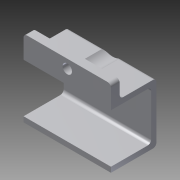
# Autodesk Inventor part: capot
Saved by Autodesk Inventor 2014 SP2 (Build 180246200, 246)
## iProperties
Created: 2015-03-19
Part Number: capot
Material: Plastique ABS
Document SubType Name: Modeling
Designer: sd
Density: 1.06 g/cm^3
Appearance: Lisse - Blanc
Mass: 7.9235 g
Surface Area: 23.98 cm^2
Volume: 7.475 cm^3
Author: sd
Autodesk Inventor part; units mm, degrees
ref_plane "YZ Plane" through (0, 0, 0) normal (1, 0, 0) x (0, 1, 0)
ref_plane "XZ Plane" through (0, 0, 0) normal (0, 1, 0) x (-1, 0, 0)
ref_plane "XY Plane" through (0, 0, 0) normal (0, 0, 1) x (1, 0, 0)
sketch "Esquisse1" plane through (0, 0, 0) normal (0, 1, 0) x (-1, 0, 0)
  line L0 (-12.5, 11) -> (12.5, 11)
  line L1 (12.5, 11) -> (12.5, -11)
  line L2 (12.5, -11) -> (-12.5, -11)
  line L3 (-12.5, -11) -> (-12.5, 11)
  point P0 (0, 0)
  dimension "d0" = 25
  dimension "d1" = 22
  dimension "d2" = 11
  dimension "d3" = 12.5
  constraints: 8 end point, 2 parallel, 1 horizontal, 1 perpendicular
  measures "d0" distance of L0.start L0.end
  measures "d1" distance of L2.end L0.start
  measures "d2" vertical distance of point (0, 0) L0.start
  measures "d3" horizontal distance of point (0, 0) L0.start
extrude "Extrusion1" add sketch "Esquisse1" along normal blind 13
sketch "Esquisse2" plane through (0, 13, 0) normal (0, 1, 0) x (1, 0, 0)
  line L0 (-12.5, 11) -> (-12.5, -11) projected
  line L1 (-12.5, -6) -> (12.5, -6)
  line L2 (12.5, -6) -> (12.5, -11)
  line L3 (12.5, -11) -> (-12.5, -11)
  line L4 (-12.5, -11) -> (-12.5, -6)
  point P0 (0, 0)
  dimension "d6" = 5
  constraints: 8 end point, 2 parallel, 1 horizontal, 1 perpendicular, 1 point on line
  measures "d6" distance of L3.end L1.start
extrude "Extrusion3" cut sketch "Esquisse2" against normal blind 10.5
fillet "Congé2" radius 1 1 edges at (0, 2.5, 6)
sketch "Esquisse4" plane through (0, 13, 0) normal (0, 1, 0) x (1, 0, 0)
  circle A0 centre (0, -8.5) radius 3.5
  line L0 (12.5, -11) -> (-12.5, -11) projected
  point P0 (12.5, -6)
  point P1 (0, 0)
  dimension "d11" = 7
  dimension "d12" = 2.5
  dimension "d13" = 5
  constraints: 1 centre point
  measures "d11" diameter of A0
  measures "d12" distance from line of L0 A0.centre
  measures "d13" distance of L0.start point (12.5, -6)
extrude "Extrusion4" cut sketch "Esquisse4" against normal blind 10.5
sketch "Esquisse6" plane through (0, 0, 0) normal (0, -1, 0) x (1, 0, 0)
  line L0 (-12.5, 11) -> (-12.5, -11) projected
  line L1 (-12.5, -11) -> (12.5, -11) projected
  line L2 (12.5, -11) -> (12.5, 11) projected
  line L3 (-12.5, -9.5) -> (12.5, -9.5)
  line L4 (12.5, -9.5) -> (12.5, 4.5)
  line L5 (12.5, 4.5) -> (-12.5, 4.5)
  line L6 (-12.5, 4.5) -> (-12.5, -9.5)
  point P0 (0, 0)
  dimension "d17" = 0
  dimension "d18" = 0
  dimension "d19" = 1.5
  dimension "d20" = 6.5
  constraints: 8 end point, 2 parallel, 1 horizontal, 1 perpendicular
  measures "d17" distance between parallel lines of L0 L6
  measures "d18" distance between parallel lines of L2 L4
  measures "d19" distance between parallel lines of L1 L3
  measures "d20" distance of L5.end L0.start
extrude "Extrusion5" cut sketch "Esquisse6" against normal blind 11.5 contours L5 L2 L3 L0
fillet "Congé3" radius 1 2 edges at (-12.5, 1.25, 11) (12.5, 1.25, 11)
fillet "Congé4" radius 1 5 edges at (0, 11.5, -9.5) (0, 13, -11) (0, 11.5, 4.5) (-7.4747, 13, 6) (7.4747, 13, 6)
sketch "Esquisse7" plane through (0, 2.5, 0) normal (0, 1, 0) x (1, 0, 0)
  arc A0 (3.1623, -7) -> (-3.1623, -7) centre (0, -8.5) ccw projected
  circle A1 centre (0, -8.5) radius 1.35
  point P0 (0, 0)
  dimension "d27" = 2.7
  constraints: 1 centre point, 1 coincident
  measures "d27" diameter of A1
extrude "Extrusion6" cut sketch "Esquisse7" against normal through all
equation "\"d2\" = 0.5 * d1"
equation "\"d3\" = 0.5 * d0"
equation "\"d12\" = 0.5 * d13"
